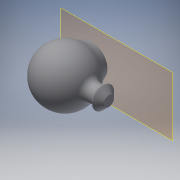
# Autodesk Inventor part: The Thing
Saved by Autodesk Inventor 2017 (Build 210142000, 142)
## iProperties
Created: 2017-03-09
Part Number: The Thing
Material: Generic
Document SubType Name: Modeling
Designer: PLTW
Density: 1 g/cm^3
Appearance: Default
Author: PLTW
Autodesk Inventor part; units mm, degrees
ref_plane "YZ Plane" through (0, 0, 0) normal (1, 0, 0) x (0, 1, 0)
ref_plane "XZ Plane" through (0, 0, 0) normal (0, 1, 0) x (-1, 0, 0)
sketch "Sketch3" plane through (0, 0, 0) normal (0, 0, 1) x (1, 0, 0)
  line L0 (-10.8841, 4.3559) -> (-10.16, 5.08)
  line L1 (-10.16, 5.08) -> (-7.62, 2.54)
  line L2 (-7.62, 2.54) -> (-7.62, -2.54)
  line L3 (-7.62, -2.54) -> (-10.16, -5.08)
  line L4 (-10.16, -5.08) -> (-10.8841, -4.3559)
  line L5 (-10.8912, 3.81) -> (-9.525, 5.1762)
  line L6 (-9.525, 5.1762) -> (-6.731, 2.3822)
  line L7 (-6.731, 2.3822) -> (-6.731, 0)
  line L8 (-6.731, 0) -> (-17.2412, 0)
  line L9 (-10.8912, 3.81) -> (-17.2412, 3.81)
  line L10 (-17.2412, 3.81) -> (-17.2412, 0)
  line L11 (-6.35, 2.54) -> (-6.35, -2.54)
  line L12 (-9.525, 5.715) -> (-6.35, 2.54)
  line L13 (-10.8841, 4.3559) -> (-9.525, 5.715)
  line L14 (-6.35, -2.54) -> (-9.525, -5.715)
  line L15 (-9.525, -5.715) -> (-10.8841, -4.3559)
  point P0 (0, 0)
  point P1 (-7.62, 0)
  dimension "d5" = 0.381
  dimension "d12" = 6.35
  dimension "d13" = 3.81
  dimension "d24" = 0.381
  dimension "d25" = 0.381
  constraints: 32 end point, 3 parallel, 3 perpendicular, 3 vertical, 1 horizontal, 1 horizontal alignment, 1 midpoint, 28 other
  measures "d5" distance between parallel lines of L0 L5
  measures "d12" distance of L5.start L9.end
  measures "d13" distance of L9.end L8.end
  measures "d24" distance between parallel lines of L12 L6
  measures "d25" distance between parallel lines of L11 L7
revolve "Revolution2" add sketch "Sketch3" angle 360 about axis through (-6.731, 0, 0) along (-1, 0, 0) contours L5 L6 L7 L8 L2 L1 | L1 L2 L8 L10 L9 L5
fillet "Fillet2" radius 0.127 3 edges at (-9.525, -5.1762, 0) (-10.8912, -3.81, 0) (-6.731, -2.3822, 0)
sketch "Sketch5" plane through (0, 0, 0) normal (0, 1, 0) x (-1, 0, 0)
  line L0 (17.2412, 3.81) -> (17.2412, -3.81) projected
  line L1 (17.2412, 3.81) -> (17.2412, -3.81) projected
  line L2 (10.9438, 3.81) -> (10.9438, -3.81) projected
  arc A0 (27.4012, 12.7) -> (27.4012, -12.7) centre (27.4012, 0) ccw
  line L3 (27.4012, 12.7) -> (27.4012, -12.7)
  point P0 (0, 0)
  dimension "d14" = 25.4
  dimension "d15" = 2.54
  constraints: 3 point on circle, 2 end point, 2 vertical alignment, 1 centre point, 1 horizontal alignment, 1 vertical
  measures "d14" distance of L3.end A0.start
  measures "d15" distance edge to line of A0 L0
revolve "Revolution3" add sketch "Sketch5" angle 360 about axis through (-27.4012, 0, 12.7) along (0, 0, -1)
ref_plane "Work Plane1" through (0, 0, -12.7) normal (0, 0, 1) x (1, 0, 0)
sketch "Sketch8" plane through (0, 0, -12.7) normal (0, 0, 1) x (1, 0, 0)
  line L0 (-15.2862, -3.81) -> (-15.2862, 3.81) projected
  circle A0 centre (-27.7622, 0) radius 7.62
  point P0 (0, 0)
  dimension "d18" = 27.7622
  dimension "d19" = 15.24
  constraints: 1 centre point, 1 coincident, 1 horizontal alignment
  measures "d18" distance of point (-27.762, 0) point (0, 0)
  measures "d19" diameter of A0
extrude "Extrusion1" add sketch "Sketch8" along normal up to next
fillet "Fillet3" radius 12.7 1 edges at (-35.3822, 0.0025, -9.8789)
fillet "Fillet4" radius 3.175 3 edges at (-15.2862, -3.81, 0) (-15.2862, 2.6939, 2.6943) (-15.2862, 2.6939, -2.6943)
equation "\"d24\" = d5"
equation "\"d25\" = d5"
body "Solid2"
